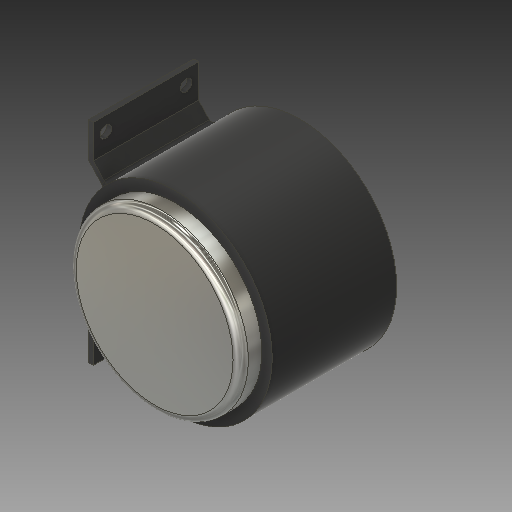
# Autodesk Inventor part: motor
Saved by Autodesk Inventor 2019 (Build 230136000, 136)
## iProperties
Created: 2017-10-27
Part Number: motor
Material: Generic
Document SubType Name: Modeling
Designer: Ajay.J
Density: 1 g/cm^3
Appearance: Steel
Author: Ajay.J
Autodesk Inventor part; units mm, degrees
ref_plane "YZ Plane" through (0, 0, 0) normal (1, 0, 0) x (0, 1, 0)
ref_plane "XZ Plane" through (0, 0, 0) normal (0, 1, 0) x (-1, 0, 0)
ref_plane "XY Plane" through (0, 0, 0) normal (0, 0, 1) x (1, 0, 0)
sketch "Sketch1" plane through (0, 0, 0) normal (0, 0, 1) x (1, 0, 0)
  circle A0 centre (0, 0) radius 50.5
  dimension "d0" = 101
  constraints: 1 centre point, 1 coincident
  measures "d0" diameter of A0
sketch "Sketch1 outline for Extrusion1" plane through (0, 0, 0) normal (0, 0, 1) x (1, 0, 0)
  circle A0 centre (0, 0) radius 50.5
extrude "Extrusion1" add sketch "Sketch1 outline for Extrusion1" along normal mid plane 65
sketch "Sketch2" plane through (0, 0, 32.5) normal (0, 0, 1) x (1, 0, 0)
  circle A0 centre (0, 0) radius 45
  dimension "d3" = 90
  constraints: 1 centre point, 1 coincident
  measures "d3" diameter of A0
sketch "Sketch2 outline for Extrusion2" plane through (0, 0, 32.5) normal (0, 0, 1) x (1, 0, 0)
  circle A0 centre (0, 0) radius 45
extrude "Extrusion2" add sketch "Sketch2 outline for Extrusion2" along normal blind 11 separate body
sketch "Sketch3" plane through (0, 0, -32.5) normal (0, 0, -1) x (-1, 0, 0)
  circle A0 centre (0, 0) radius 45
  dimension "d6" = 90
  constraints: 1 centre point, 1 coincident
  measures "d6" diameter of A0
sketch "Sketch3 outline for Extrusion3" plane through (0, 0, -32.5) normal (0, 0, -1) x (-1, 0, 0)
  circle A0 centre (0, 0) radius 45
extrude "Extrusion3" add sketch "Sketch3 outline for Extrusion3" along normal blind 5 bodies 1
sketch "Sketch4" plane through (0, 0, 0) normal (0, 0, 1) x (1, 0, 0)
  line L0 (-50.5, 36.598952) -> (-50.5, 55)
  line L1 (-50.5, 55) -> (-48, 55)
  line L2 (-48, 55) -> (-48, 37.569428)
  line L3 (-48, 37.569428) -> (-40.826794, 29.72243)
  circle A0 centre (0, 0) radius 50.5
  line L4 (-50.5, 36.598952) -> (-42.283548, 27.610714)
  dimension "d9" = 55
  dimension "d10" = 2.5
  dimension "d11" = 2.5
  dimension "d12" = 18.40105
  dimension "d13" = 17.43057
  constraints: 10 end point, 2 perpendicular, 2 point on circle, 1 parallel, 1 tangent, 1 vertical
  measures "d9" distance from line of point (0, 0) L1
  measures "d10" distance between parallel lines of L0 L2
  measures "d11" distance between parallel lines of L4 L3
  measures "d12" distance of L0.start L0.end
  measures "d13" distance of L1.end L2.end
sketch "Sketch4 outline for Extrusion4" plane through (0, 0, 0) normal (0, 0, 1) x (1, 0, 0)
  line L0 (-50.5, 55) -> (-50.5, 36.598952)
  line L1 (-48, 55) -> (-50.5, 55)
  line L2 (-48, 37.569428) -> (-48, 55)
  line L3 (-40.826794, 29.72243) -> (-48, 37.569428)
  arc A0 (-42.283548, 27.610714) -> (-40.826794, 29.72243) centre (0, 0) cw
  line L4 (-50.5, 36.598952) -> (-42.283548, 27.610714)
extrude "Extrusion4" add sketch "Sketch4 outline for Extrusion4" along normal mid plane 55 bodies 1
mirror "Mirror1" about plane through (0, 0, 0) normal (0, 1, 0) of "Extrusion4" bodies 1
sketch "Sketch5" plane through (-50.5, 36.598952, 27.5) normal (-1, 0, 0) x (0, 0, 1)
  line L0 (-27.5, 52.121928) -> (-27.5, -131.017503) construction
  point P0 (-27.5, -36.598952)
  point P1 (-6.5, 10.901048)
  point P2 (-48.5, 10.901048)
  dimension "d16" = 42
  dimension "d17" = 47.5
  constraints: 2 end point, 1 point on line, 1 symmetric about line, 1 vertical
  measures "d16" distance of point (-48.5, 10.901) point (-6.5, 10.901)
  measures "d17" vertical distance of point (-27.5, -36.599) point (-48.5, 10.901)
hole "Hole1" at (-50.5, 47.5, 21) at (-50.5, 47.5, -21) direction (1, 0, 0) diameter 6 depth 4.825 bodies 1
mirror "Mirror2" about plane through (0, 0, 0) normal (0, 1, 0) of "Hole1" bodies 1
sketch "Sketch6" plane through (0, 0, -37.5) normal (0, 0, -1) x (-1, 0, 0)
  point P0 (0, 0)
sketch "Sketch7" plane through (0, 0, -37.5) normal (0, 0, -1) x (-1, 0, 0)
  circle A0 centre (0, 0) radius 5
  dimension "d25" = 10
  constraints: 1 centre point, 1 coincident
  measures "d25" diameter of A0
sketch "Sketch7 outline for Extrusion5" plane through (0, 0, -37.5) normal (0, 0, -1) x (-1, 0, 0)
  circle A0 centre (0, 0) radius 5
extrude "Extrusion5" add sketch "Sketch7 outline for Extrusion5" along normal blind 25 separate body
fillet "Fillet1" radius 4 1 edges at (-45, 0, 43.5)
fillet "Fillet3" radius 2 8 edges at (-42.2835, 27.6107, 0) (-40.8268, -29.7224, 0) (-42.2835, -27.6107, 0) (-40.8268, 29.7224, 0) (-41.5686, 28.6758, 27.5) (-41.5686, -28.6758, 27.5) (-41.5686, 28.6758, -27.5) (-41.5686, -28.6758, -27.5)
fillet "Fillet4" radius 2 1 edges at (45, 0, -37.5)
body "Solid1"
body "Solid2"
body "Solid3"
